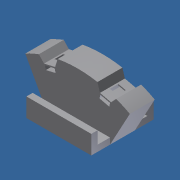
# Autodesk Inventor part: IR Sensor Piece Ver 2
Saved by Autodesk Inventor 2012 (Build 160160000, 160)
## iProperties
Created: 2012-03-08
Part Number: IR Sensor Piece Ver 2
Material: Default
Document SubType Name: Modeling
Designer: Allison Garza
Density: 1 g/cm^3
Author: Allison Garza
Autodesk Inventor part; units mm, degrees
ref_plane "YZ Plane" through (0, 0, 0) normal (1, 0, 0) x (0, 1, 0)
ref_plane "XZ Plane" through (0, 0, 0) normal (0, 1, 0) x (-1, 0, 0)
ref_plane "XY Plane" through (0, 0, 0) normal (0, 0, 1) x (1, 0, 0)
sketch "Sketch1" plane through (0, 0, 0) normal (0, 0, 1) x (1, 0, 0)
  line L0 (-46.8353, 30.48) -> (46.8353, 30.48)
  arc A0 (0, 55.88) -> (-46.8353, 30.48) centre (0, 0) ccw
  arc A1 (46.8353, 30.48) -> (0, 55.88) centre (0, 0) ccw
  constraints: 4 point on circle, 2 centre point, 2 end point, 1 coincident, 1 horizontal
extrude "Extrusion1" add sketch "Sketch1" against normal blind 12.7
sketch "Sketch2" plane through (0, 0, 0) normal (0, 0, 1) x (1, 0, 0)
  line L0 (-46.8353, 30.48) -> (46.8353, 30.48) projected
  arc A0 (46.8353, 30.48) -> (-46.8353, 30.48) centre (0, 0) ccw projected
  line L1 (0, 55.88) -> (0, 0)
  line L2 (0, 0) -> (46.8353, 30.48)
  line L3 (-46.8353, 30.48) -> (0, 0)
  line L4 (0, 0) -> (-26.6416, 49.1203)
  line L5 (0, 0) -> (26.6416, 49.1203)
  line L6 (-16.5866, 48.9387) -> (-20.0564, 52.6491)
  line L7 (-20.0564, 52.6491) -> (-18.578, 57.5092)
  line L8 (-18.578, 57.5092) -> (-13.6298, 58.659)
  line L9 (-13.6298, 58.659) -> (-10.16, 54.9486)
  line L10 (-10.16, 54.9486) -> (-11.6384, 50.0885)
  line L11 (-11.6384, 50.0885) -> (-16.5866, 48.9387)
  line L12 (16.5866, 48.9387) -> (11.6384, 50.0885)
  line L13 (11.6384, 50.0885) -> (10.16, 54.9486)
  line L14 (10.16, 54.9486) -> (13.6298, 58.659)
  line L15 (13.6298, 58.659) -> (18.578, 57.5092)
  line L16 (18.578, 57.5092) -> (20.0564, 52.6491)
  line L17 (20.0564, 52.6491) -> (16.5866, 48.9387)
  line L18 (11.6384, 50.0885) -> (16.5866, 48.9387)
  line L19 (16.5866, 48.9387) -> (16.1555, 47.0836)
  line L20 (16.1555, 47.0836) -> (11.2073, 48.2333)
  line L21 (11.2073, 48.2333) -> (11.6384, 50.0885)
  line L22 (-16.5866, 48.9387) -> (-11.6384, 50.0885)
  line L23 (-11.6384, 50.0885) -> (-11.2072, 48.2329)
  line L24 (-11.2072, 48.2329) -> (-16.1554, 47.0832)
  line L25 (-16.1554, 47.0832) -> (-16.5866, 48.9387)
  line L26 (-17.0874, 49.4743) -> (-11.425, 50.79)
  line L27 (11.425, 50.79) -> (17.0874, 49.4743)
  point P0 (-15.1082, 53.7989)
  point P1 (15.1082, 53.7989)
  dimension "d8" = 28.47
  dimension "d9" = 28.47
  dimension "d18" = 5.08
  dimension "d19" = 5.08
  dimension "d20" = 10.16
  dimension "d21" = 10.16
  dimension "d22" = 1.905
  dimension "d23" = 1.9046
  dimension "d24" = 0.635
  dimension "d25" = 0.635
  constraints: 54 end point, 6 equal length, 5 perpendicular, 4 point on line, 34 other
  measures "d8" angle of L5 L2
  measures "d9" angle of L4 L3
  measures "d18" distance of L7.end L8.end
  measures "d19" distance of L14.end L15.end
  measures "d20" horizontal distance of L1.start L13.end
  measures "d21" horizontal distance of L9.end L1.start
  measures "d22" distance of L10.end L23.end
  measures "d23" distance of L20.end L12.end
  measures "d24" distance between parallel lines of L26 L11
  measures "d25" distance between parallel lines of L27 L12
extrude "Extrusion2" cut sketch "Sketch2" against normal blind 12.7 contours A0 L4 L0 | L0 L4 L3 | L5 L0 L2 | L6 L7 L8 L9 A0 | A0 L10 L26 L6 | L0 L5 A0 | L14 L15 L16 L17 A0 | A0 L17 L27 L13 | L11 L23 L24 L25 | L12 L19 L20 L21
sketch "Sketch3" plane through (-17.0874, 49.4743, 0) normal (-0.2263272, 0.9740513, 0) x (0.9740513, 0.2263272, 0)
  line L0 (0, 0) -> (0, 12.7) projected
  line L1 (1.0016, 8.763) -> (1.0016, 4.4937)
  line L2 (1.0016, 4.4937) -> (4.8116, 4.4937)
  line L3 (4.8116, 4.4937) -> (4.8116, 8.763)
  line L4 (4.8116, 8.763) -> (1.0016, 8.763)
  point P0 (5.8132, 12.7)
  point P1 (5.4466, 0)
  dimension "d28" = 0.635
  dimension "d29" = 3.81
  dimension "d30" = 3.937
  constraints: 8 end point, 3 parallel, 1 perpendicular
  measures "d28" horizontal distance of point (5.447, 0) L2.end
  measures "d29" distance of L3.end L1.start
  measures "d30" vertical distance of point (5.813, 12.7) L3.end
extrude "Extrusion3" cut sketch "Sketch3" against normal up to next
sketch "Sketch4" plane through (11.425, 50.79, 0) normal (0.2263272, 0.9740513, 0) x (0.9740513, -0.2263272, 0)
  line L0 (0, 0) -> (0, 12.7) projected
  line L1 (0.635, 8.763) -> (0.635, 4.4958)
  line L2 (0.635, 4.4958) -> (4.445, 4.4958)
  line L3 (4.445, 4.4958) -> (4.445, 8.763)
  line L4 (4.445, 8.763) -> (0.635, 8.763)
  point P0 (0.3666, 0)
  dimension "d33" = 3.81
  dimension "d34" = 3.937
  dimension "d35" = 0.635
  dimension "d36" = 4.2672
  constraints: 8 end point, 3 parallel, 1 perpendicular
  measures "d33" distance of L3.end L1.start
  measures "d34" vertical distance of L0.end L1.start
  measures "d35" horizontal distance of L0.start L1.end
  measures "d36" distance of L1.start L1.end
extrude "Extrusion4" cut sketch "Sketch4" against normal up to next
sketch "Sketch5" plane through (0, 0, -12.7) normal (0, 0, -1) x (-1, 0, 0)
  line L0 (16.5316, 30.48) -> (-16.5316, 30.48) projected
  line L1 (-16.5316, 30.48) -> (16.5316, 30.48)
  line L2 (16.5316, 30.48) -> (16.5316, 33.655)
  line L3 (16.5316, 33.655) -> (-16.5316, 33.655)
  line L4 (-16.5316, 33.655) -> (-16.5316, 30.48)
  dimension "d39" = 3.175
  constraints: 8 end point, 3 equal length, 1 perpendicular
  measures "d39" distance of L0.start L2.end
extrude "Extrusion5" add sketch "Sketch5" along normal blind 9.525
sketch "Sketch7" plane through (-16.5316, 33.655, -12.7) normal (0, 1, 0) x (1, 0, 0)
  line L0 (33.0631, 9.525) -> (0, 9.525) projected
  line L1 (0, 9.525) -> (33.0631, 9.525)
  line L2 (33.0631, 9.525) -> (33.0631, 6.35)
  line L3 (33.0631, 6.35) -> (0, 6.35)
  line L4 (0, 6.35) -> (0, 9.525)
  point P0 (16.5316, -12.7)
  dimension "d42" = 3.175
  constraints: 8 end point, 3 equal length, 1 perpendicular
  measures "d42" distance of L0.start L2.end
extrude "Extrusion6" add sketch "Sketch7" along normal blind 6.35
sketch "Sketch8" plane through (0, 0, 0) normal (0, 0, 1) x (1, 0, 0)
  line L0 (-16.5316, 30.48) -> (16.5316, 30.48) projected
  line L1 (-16.5316, 30.48) -> (16.5316, 30.48)
  line L2 (16.5316, 30.48) -> (16.5316, 33.655)
  line L3 (16.5316, 33.655) -> (-16.5316, 33.655)
  line L4 (-16.5316, 33.655) -> (-16.5316, 30.48)
  dimension "d45" = 3.175
  constraints: 8 end point, 3 equal length, 1 perpendicular
  measures "d45" distance of L0.end L2.end
extrude "Extrusion7" add sketch "Sketch8" along normal blind 9.525
sketch "Sketch9" plane through (-16.5316, 33.655, 0) normal (0, 1, 0) x (1, 0, 0)
  line L0 (0, -9.525) -> (33.0631, -9.525) projected
  line L1 (0, -9.525) -> (33.0631, -9.525)
  line L2 (33.0631, -9.525) -> (33.0631, -6.35)
  line L3 (33.0631, -6.35) -> (0, -6.35)
  line L4 (0, -6.35) -> (0, -9.525)
  point P0 (16.5316, 0)
  dimension "d48" = 3.175
  constraints: 8 end point, 3 equal length, 1 perpendicular
  measures "d48" distance of L0.end L2.end
extrude "Extrusion8" add sketch "Sketch9" along normal blind 6.35
body "Solid1"
